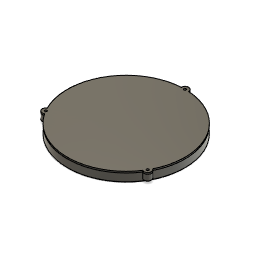
charging_base (Autodesk Fusion 360 design; units mm, degrees)
Autodesk Fusion 360 part; units mm, degrees
sketch "Sketch1" plane through (0, 0, 0) normal (0, 1, 0) x (1, 0, 0)
  circle A0 centre (0, 0) radius 65
  dimension "d1" = 130
  constraint coincident A0.centre origin
  measures "d1" diameter of A0
extrude "Extrude1" add sketch "Sketch1" along normal blind 1.6 makes body 1
sketch "Sketch2" plane through (0, 1.6, 0) normal (0, 1, 0) x (-1, 0, 0)
  circle A0 centre (0, 0) radius 65
  circle A1 centre (0, 0) radius 65
  circle A2 centre (0, 0) radius 62.5
  dimension "d4" = 130
  dimension "d5" = 125
  constraint coincident A0.centre A1.centre
  measures "d4" diameter of A1
  measures "d5" diameter of A2
extrude "Extrude2" add sketch "Sketch2" along normal blind 6.2 bodies 1
sketch "Sketch3" plane through (0, 1.6, 0) normal (0, 1, 0) x (-1, 0, 0)
  circle A0 centre (0, 0) radius 62.5
  circle A1 centre (0, 0) radius 20
  line L0 (0, 0) -> (0.5, 0)
  line L1 (0.5, 0) -> (-0.5, 0)
  circle A2 centre (0, 0) radius 62.5
  line L2 (-0.5, -47.9974) -> (-0.5, -62.498)
  line L3 (0.5, -62.498) -> (0.5, -47.9974)
  line L4 (0.5, -46.9973) -> (0.5, -33.9963)
  line L5 (0.5, -32.9962) -> (0.5, -20.994)
  line L6 (-0.5, -20.994) -> (-0.5, -32.9962)
  line L7 (-0.5, -33.9963) -> (-0.5, -46.9973)
  arc A3 (0.5, -47.9974) -> (23.5657, -41.817) centre (0, 0) ccw
  arc A4 (0.5, -46.9973) -> (23.0657, -40.9509) centre (0, 0) ccw
  line L8 (31.682, -53.8749) -> (24.4317, -41.317)
  line L9 (23.5657, -41.817) -> (30.816, -54.3749)
  arc A5 (0.5, -33.9963) -> (16.5651, -29.6917) centre (0, 0) ccw
  arc A6 (0.5, -32.9962) -> (16.0651, -28.8256) centre (0, 0) ccw
  line L10 (23.9317, -40.4509) -> (17.4312, -29.1917)
  line L11 (16.9311, -28.3256) -> (10.93, -17.9314)
  line L12 (10.064, -18.4314) -> (16.0651, -28.8256)
  line L13 (16.5651, -29.6917) -> (23.0657, -40.9509)
  arc A7 (0.5, -20.994) -> (10.064, -18.4314) centre (0, 0) ccw
  arc A8 (-10.064, -18.4314) -> (-0.5, -20.994) centre (0, 0) ccw
  arc A9 (-16.0651, -28.8256) -> (-0.5, -32.9962) centre (0, 0) ccw
  arc A10 (-16.5651, -29.6917) -> (-0.5, -33.9963) centre (0, 0) ccw
  line L14 (-16.0651, -28.8256) -> (-10.064, -18.4314)
  line L15 (-10.93, -17.9314) -> (-16.9311, -28.3256)
  arc A11 (-23.0657, -40.9509) -> (-0.5, -46.9973) centre (0, 0) ccw
  arc A12 (-23.5657, -41.817) -> (-0.5, -47.9974) centre (0, 0) ccw
  line L16 (-30.816, -54.3749) -> (-23.5657, -41.817)
  line L17 (-23.0657, -40.9509) -> (-16.5651, -29.6917)
  line L18 (-17.4312, -29.1917) -> (-23.9317, -40.4509)
  line L19 (-24.4317, -41.317) -> (-31.682, -53.8749)
  line L20 (41.317, -24.4317) -> (53.8749, -31.682)
  arc A13 (23.9317, -40.4509) -> (40.4509, -23.9317) centre (0, 0) ccw
  arc A14 (24.4317, -41.317) -> (41.317, -24.4317) centre (0, 0) ccw
  line L21 (54.3749, -30.816) -> (41.817, -23.5657)
  line L22 (17.9314, -10.93) -> (28.3256, -16.9311)
  line L23 (29.1917, -17.4312) -> (40.4509, -23.9317)
  line L24 (40.9509, -23.0657) -> (29.6917, -16.5651)
  line L25 (28.8256, -16.0651) -> (18.4314, -10.064)
  arc A15 (16.9311, -28.3256) -> (28.3256, -16.9311) centre (0, 0) ccw
  arc A16 (17.4312, -29.1917) -> (29.1917, -17.4312) centre (0, 0) ccw
  arc A17 (10.93, -17.9314) -> (17.9314, -10.93) centre (0, 0) ccw
  arc A18 (18.4314, -10.064) -> (20.994, -0.5) centre (0, 0) ccw
  arc A19 (28.8256, -16.0651) -> (32.9962, -0.5) centre (0, 0) ccw
  arc A20 (29.6917, -16.5651) -> (33.9963, -0.5) centre (0, 0) ccw
  arc A21 (40.9509, -23.0657) -> (46.9973, -0.5) centre (0, 0) ccw
  arc A22 (41.817, -23.5657) -> (47.9974, -0.5) centre (0, 0) ccw
  arc A23 (20.994, 0.5) -> (18.4314, 10.064) centre (0, 0) ccw
  arc A24 (32.9962, 0.5) -> (28.8256, 16.0651) centre (0, 0) ccw
  arc A25 (33.9963, 0.5) -> (29.6917, 16.5651) centre (0, 0) ccw
  arc A26 (46.9973, 0.5) -> (40.9509, 23.0657) centre (0, 0) ccw
  arc A27 (47.9974, 0.5) -> (41.817, 23.5657) centre (0, 0) ccw
  line L26 (20.994, -0.5) -> (32.9962, -0.5)
  line L27 (32.9962, 0.5) -> (20.994, 0.5)
  line L28 (33.9963, -0.5) -> (46.9973, -0.5)
  line L29 (47.9974, -0.5) -> (62.498, -0.5)
  line L30 (62.498, 0.5) -> (47.9974, 0.5)
  line L31 (46.9973, 0.5) -> (33.9963, 0.5)
  line L32 (18.4314, 10.064) -> (28.8256, 16.0651)
  line L33 (28.3256, 16.9311) -> (17.9314, 10.93)
  line L34 (29.6917, 16.5651) -> (40.9509, 23.0657)
  line L35 (41.817, 23.5657) -> (54.3749, 30.816)
  line L36 (53.8749, 31.682) -> (41.317, 24.4317)
  line L37 (40.4509, 23.9317) -> (29.1917, 17.4312)
  arc A28 (17.9314, 10.93) -> (10.93, 17.9314) centre (0, 0) ccw
  arc A29 (28.3256, 16.9311) -> (16.9311, 28.3256) centre (0, 0) ccw
  arc A30 (29.1917, 17.4312) -> (17.4312, 29.1917) centre (0, 0) ccw
  arc A31 (40.4509, 23.9317) -> (23.9317, 40.4509) centre (0, 0) ccw
  arc A32 (41.317, 24.4317) -> (24.4317, 41.317) centre (0, 0) ccw
  arc A33 (10.064, 18.4314) -> (0.5, 20.994) centre (0, 0) ccw
  arc A34 (16.0651, 28.8256) -> (0.5, 32.9962) centre (0, 0) ccw
  arc A35 (16.5651, 29.6917) -> (0.5, 33.9963) centre (0, 0) ccw
  arc A36 (23.0657, 40.9509) -> (0.5, 46.9973) centre (0, 0) ccw
  arc A37 (23.5657, 41.817) -> (0.5, 47.9974) centre (0, 0) ccw
  line L38 (10.93, 17.9314) -> (16.9311, 28.3256)
  line L39 (16.0651, 28.8256) -> (10.064, 18.4314)
  line L40 (17.4312, 29.1917) -> (23.9317, 40.4509)
  line L41 (24.4317, 41.317) -> (31.682, 53.8749)
  line L42 (30.816, 54.3749) -> (23.5657, 41.817)
  line L43 (23.0657, 40.9509) -> (16.5651, 29.6917)
  line L44 (0.5, 20.994) -> (0.5, 32.9962)
  line L45 (-0.5, 32.9962) -> (-0.5, 20.994)
  line L46 (0.5, 33.9963) -> (0.5, 46.9973)
  line L47 (0.5, 47.9974) -> (0.5, 62.498)
  line L48 (-0.5, 62.498) -> (-0.5, 47.9974)
  line L49 (-0.5, 46.9973) -> (-0.5, 33.9963)
  arc A38 (-0.5, 20.994) -> (-10.064, 18.4314) centre (0, 0) ccw
  arc A39 (-0.5, 32.9962) -> (-16.0651, 28.8256) centre (0, 0) ccw
  arc A40 (-0.5, 33.9963) -> (-16.5651, 29.6917) centre (0, 0) ccw
  arc A41 (-0.5, 46.9973) -> (-23.0657, 40.9509) centre (0, 0) ccw
  arc A42 (-0.5, 47.9974) -> (-23.5657, 41.817) centre (0, 0) ccw
  line L50 (-10.064, 18.4314) -> (-16.0651, 28.8256)
  line L51 (-16.9311, 28.3256) -> (-10.93, 17.9314)
  line L52 (-16.5651, 29.6917) -> (-23.0657, 40.9509)
  line L53 (-23.5657, 41.817) -> (-30.816, 54.3749)
  line L54 (-31.682, 53.8749) -> (-24.4317, 41.317)
  line L55 (-23.9317, 40.4509) -> (-17.4312, 29.1917)
  arc A43 (-10.93, 17.9314) -> (-17.9314, 10.93) centre (0, 0) ccw
  arc A44 (-16.9311, 28.3256) -> (-28.3256, 16.9311) centre (0, 0) ccw
  arc A45 (-17.4312, 29.1917) -> (-29.1917, 17.4312) centre (0, 0) ccw
  arc A46 (-23.9317, 40.4509) -> (-40.4509, 23.9317) centre (0, 0) ccw
  arc A47 (-24.4317, 41.317) -> (-41.317, 24.4317) centre (0, 0) ccw
  line L56 (-17.9314, 10.93) -> (-28.3256, 16.9311)
  line L57 (-28.8256, 16.0651) -> (-18.4314, 10.064)
  line L58 (-29.1917, 17.4312) -> (-40.4509, 23.9317)
  line L59 (-41.317, 24.4317) -> (-53.8749, 31.682)
  line L60 (-54.3749, 30.816) -> (-41.817, 23.5657)
  line L61 (-40.9509, 23.0657) -> (-29.6917, 16.5651)
  arc A48 (-18.4314, 10.064) -> (-20.994, 0.5) centre (0, 0) ccw
  arc A49 (-28.8256, 16.0651) -> (-32.9962, 0.5) centre (0, 0) ccw
  arc A50 (-29.6917, 16.5651) -> (-33.9963, 0.5) centre (0, 0) ccw
  arc A51 (-40.9509, 23.0657) -> (-46.9973, 0.5) centre (0, 0) ccw
  arc A52 (-41.817, 23.5657) -> (-47.9974, 0.5) centre (0, 0) ccw
  line L62 (-20.994, 0.5) -> (-32.9962, 0.5)
  line L63 (-32.9962, -0.5) -> (-20.994, -0.5)
  line L64 (-33.9963, 0.5) -> (-46.9973, 0.5)
  line L65 (-47.9974, 0.5) -> (-62.498, 0.5)
  line L66 (-62.498, -0.5) -> (-47.9974, -0.5)
  line L67 (-46.9973, -0.5) -> (-33.9963, -0.5)
  arc A53 (-20.994, -0.5) -> (-18.4314, -10.064) centre (0, 0) ccw
  arc A54 (-17.9314, -10.93) -> (-10.93, -17.9314) centre (0, 0) ccw
  arc A55 (-32.9962, -0.5) -> (-28.8256, -16.0651) centre (0, 0) ccw
  arc A56 (-28.3256, -16.9311) -> (-16.9311, -28.3256) centre (0, 0) ccw
  arc A57 (-33.9963, -0.5) -> (-29.6917, -16.5651) centre (0, 0) ccw
  arc A58 (-29.1917, -17.4312) -> (-17.4312, -29.1917) centre (0, 0) ccw
  arc A59 (-46.9973, -0.5) -> (-40.9509, -23.0657) centre (0, 0) ccw
  arc A60 (-40.4509, -23.9317) -> (-23.9317, -40.4509) centre (0, 0) ccw
  arc A61 (-47.9974, -0.5) -> (-41.817, -23.5657) centre (0, 0) ccw
  arc A62 (-41.317, -24.4317) -> (-24.4317, -41.317) centre (0, 0) ccw
  line L68 (-18.4314, -10.064) -> (-28.8256, -16.0651)
  line L69 (-28.3256, -16.9311) -> (-17.9314, -10.93)
  line L70 (-53.8749, -31.682) -> (-41.317, -24.4317)
  line L71 (-40.4509, -23.9317) -> (-29.1917, -17.4312)
  line L72 (-29.6917, -16.5651) -> (-40.9509, -23.0657)
  line L73 (-41.817, -23.5657) -> (-54.3749, -30.816)
  dimension "d8" = 40
  dimension "d9" = 42
  dimension "d10" = 0.5
  dimension "d11" = 1
  dimension "d15" = 125
  dimension "d16" = 66
  dimension "d17" = 68
  dimension "d18" = 94
  dimension "d19" = 96
  constraint coincident A0.centre A1.centre
  constraint horizontal L0
  constraint horizontal L1
  constraint vertical L6
  constraint vertical L3
  constraint coincident A0 L8.start
  constraint coincident A0 L9.end
  constraint coincident A0 L3.start
  constraint coincident A0 L2.end
  constraint coincident A0 L16.start
  constraint coincident A0 L19.end
  constraint coincident A0 L70.start
  constraint coincident A0 L73.end
  constraint coincident A0 L66.start
  constraint coincident A0 L65.end
  constraint coincident A0 L59.end
  constraint coincident A0 L60.start
  constraint coincident A0 L20.end
  constraint coincident A0 L21.start
  constraint coincident A0 L29.end
  constraint coincident A0 L30.start
  constraint coincident A0 L35.end
  constraint coincident A0 L36.start
  constraint coincident A0 L41.end
  constraint coincident A0 L42.start
  constraint coincident A0 L47.end
  constraint coincident A0 L48.start
  constraint coincident A0 L53.end
  constraint coincident A0 L54.start
  constraint coincident L2.start L6
  constraint coincident L4.start L3
  constraint collinear L2 L6
  constraint collinear L3 L4
  constraint coincident L7.start L6
  constraint collinear L4 L5
  constraint collinear L6 L7
  constraint coincident A3.end L12
  constraint concentric A3 A14
  constraint coincident L10.start L8
  constraint concentric A4 A13
  constraint collinear L8 L10
  constraint collinear L9 L12
  constraint coincident A5.end L12
  constraint concentric A5 A16
  constraint coincident L11.start L10
  constraint concentric A6 A15
  constraint collinear L10 L11
  constraint collinear L12 L13
  constraint concentric A7 A17
  constraint concentric A8 A17
  constraint coincident A9.start L16
  constraint concentric A9 A15
  constraint coincident L18.start L15
  constraint concentric A10 A16
  constraint collinear L14 L16
  constraint collinear L15 L18
  constraint coincident A11.start L16
  constraint concentric A11 A13
  constraint coincident L19.start L18
  constraint concentric A12 A14
  constraint collinear L16 L17
  constraint collinear L18 L19
  constraint collinear L20 L22
  constraint coincident L24.start L21
  constraint concentric A13 A21
  constraint concentric A14 A22
  constraint collinear L21 L24
  constraint collinear L22 L23
  constraint coincident L24.end A16
  constraint coincident L25.start A15
  constraint collinear L24 L25
  constraint concentric A15 A19
  constraint concentric A16 A20
  constraint concentric A17 A18
  constraint concentric A18 A23
  constraint coincident A24.start L30
  constraint concentric A19 A24
  constraint coincident A20.end L26
  constraint concentric A20 A25
  constraint coincident A21.end L26
  constraint coincident A26.start L30
  constraint concentric A21 A26
  constraint coincident A22.end L26
  constraint concentric A22 A27
  constraint concentric A23 A28
  constraint coincident L33.start L36
  constraint concentric A24 A29
  constraint coincident A25.end L32
  constraint concentric A25 A30
  constraint coincident A26.end L32
  constraint coincident L37.start L36
  constraint concentric A26 A31
  constraint coincident A27.end L32
  constraint concentric A27 A32
  constraint collinear L26 L28
  constraint collinear L27 L30
  constraint collinear L28 L29
  constraint collinear L30 L31
  constraint collinear L32 L34
  constraint collinear L33 L36
  constraint collinear L34 L35
  constraint collinear L36 L37
  constraint concentric A28 A33
  constraint coincident A34.start L42
  constraint concentric A29 A34
  constraint coincident A30.end L38
  constraint concentric A30 A35
  constraint coincident A31.end L38
  constraint coincident A36.start L42
  constraint concentric A31 A36
  constraint coincident A32.end L38
  constraint concentric A32 A37
  constraint concentric A33 A38
  constraint coincident L45.start L48
  constraint concentric A34 A39
  constraint coincident A35.end L44
  constraint concentric A35 A40
  constraint coincident A36.end L44
  constraint coincident L49.start L48
  constraint concentric A36 A41
  constraint coincident A37.end L44
  constraint concentric A37 A42
  constraint collinear L38 L40
  constraint collinear L39 L42
  constraint collinear L40 L41
  constraint collinear L42 L43
  constraint collinear L44 L46
  constraint collinear L45 L48
  constraint collinear L46 L47
  constraint collinear L48 L49
  constraint concentric A38 A43
  constraint coincident L51.start L54
  constraint concentric A39 A44
  constraint coincident A40.end L50
  constraint concentric A40 A45
  constraint coincident A41.end L50
  constraint coincident L55.start L54
  constraint concentric A41 A46
  constraint coincident A42.end L50
  constraint concentric A42 A47
  constraint collinear L50 L52
  constraint collinear L51 L54
  constraint collinear L52 L53
  constraint collinear L54 L55
  constraint concentric A43 A48
  constraint coincident L57.start L60
  constraint concentric A44 A49
  constraint coincident A45.end L56
  constraint concentric A45 A50
  constraint coincident A46.end L56
  constraint coincident L61.start L60
  constraint concentric A46 A51
  constraint coincident A47.end L56
  constraint concentric A47 A52
  constraint collinear L56 L58
  constraint collinear L57 L60
  constraint collinear L58 L59
  constraint collinear L60 L61
  constraint concentric A48 A53
  constraint coincident L63.start L66
  constraint concentric A49 A55
  constraint coincident A50.end L62
  constraint concentric A50 A57
  constraint coincident A51.end L62
  constraint coincident L67.start L66
  constraint concentric A51 A59
  constraint coincident A52.end L62
  constraint concentric A52 A61
  constraint collinear L62 L64
  constraint collinear L63 L66
  constraint collinear L64 L65
  constraint collinear L66 L67
  constraint concentric A53 A54
  constraint coincident A56.start L70
  constraint concentric A55 A56
  constraint coincident A57.end L68
  constraint concentric A57 A58
  constraint coincident A59.end L68
  constraint coincident A60.start L70
  constraint concentric A59 A60
  constraint coincident A61.end L68
  constraint concentric A61 A62
  constraint collinear L68 L72
  constraint collinear L69 L70
  constraint collinear L70 L71
  constraint collinear L72 L73
  measures "d8" diameter of A1
  measures "d9" diameter of A7
  measures "d10" distance of A0.centre L0.end
  measures "d11" distance of L0.end L1.end
  measures "d15" diameter of A2
  measures "d16" diameter of A6
  measures "d17" diameter of A5
  measures "d18" diameter of A4
  measures "d19" diameter of A3
extrude "Extrude3" add sketch "Sketch3" along normal blind 5.2 contours A0 A2 L2 L3 A3 L8 L9 A12 L16 L19 L20 A14 L21 A22 A27 L29 L30 L35 L36 A32 A37 L41 L42 L47 L48 A42 L53 L54 A47 L59 L60 A52 L65 L66 A61 A62 L70 L73 bodies 1
sketch "Sketch4" plane through (0, 6.8, 0) normal (0, 1, 0) x (-1, 0, 0)
  arc A0 (-40.9509, 23.0657) -> (-46.9973, 0.5) centre (0, 0) ccw
  line L0 (-40.9509, 23.0657) -> (-29.6917, 16.5651)
  arc A1 (-29.6917, 16.5651) -> (-33.9963, 0.5) centre (0, 0) ccw
  line L1 (-33.9963, 0.5) -> (-46.9973, 0.5)
  arc A2 (0.5, -46.9973) -> (23.0657, -40.9509) centre (0, 0) ccw
  line L2 (0.5, -46.9973) -> (0.5, -33.9963)
  arc A3 (0.5, -33.9963) -> (16.5651, -29.6917) centre (0, 0) ccw
  line L3 (16.5651, -29.6917) -> (23.0657, -40.9509)
  arc A4 (-16.0651, -28.8256) -> (-0.5, -32.9962) centre (0, 0) ccw
  line L4 (-16.0651, -28.8256) -> (-10.064, -18.4314)
  arc A5 (-10.064, -18.4314) -> (-0.5, -20.994) centre (0, 0) ccw
  line L5 (-0.5, -20.994) -> (-0.5, -32.9962)
  arc A6 (28.3256, 16.9311) -> (16.9311, 28.3256) centre (0, 0) ccw
  line L6 (28.3256, 16.9311) -> (17.9314, 10.93)
  arc A7 (17.9314, 10.93) -> (10.93, 17.9314) centre (0, 0) ccw
  line L7 (10.93, 17.9314) -> (16.9311, 28.3256)
  arc A8 (23.0657, 40.9509) -> (0.5, 46.9973) centre (0, 0) ccw
  line L8 (23.0657, 40.9509) -> (16.5651, 29.6917)
  arc A9 (16.5651, 29.6917) -> (0.5, 33.9963) centre (0, 0) ccw
  line L9 (0.5, 33.9963) -> (0.5, 46.9973)
  circle A10 centre (0, 0) radius 20
  arc A11 (-0.5, 32.9962) -> (-16.0651, 28.8256) centre (0, 0) ccw
  line L10 (-0.5, 32.9962) -> (-0.5, 20.994)
  arc A12 (-0.5, 20.994) -> (-10.064, 18.4314) centre (0, 0) ccw
  line L11 (-10.064, 18.4314) -> (-16.0651, 28.8256)
  arc A13 (-46.9973, -0.5) -> (-40.9509, -23.0657) centre (0, 0) ccw
  line L12 (-46.9973, -0.5) -> (-33.9963, -0.5)
  arc A14 (-33.9963, -0.5) -> (-29.6917, -16.5651) centre (0, 0) ccw
  line L13 (-29.6917, -16.5651) -> (-40.9509, -23.0657)
  arc A15 (-23.9317, 40.4509) -> (-40.4509, 23.9317) centre (0, 0) ccw
  line L14 (-23.9317, 40.4509) -> (-17.4312, 29.1917)
  arc A16 (-17.4312, 29.1917) -> (-29.1917, 17.4312) centre (0, 0) ccw
  line L15 (-29.1917, 17.4312) -> (-40.4509, 23.9317)
  arc A17 (-40.4509, -23.9317) -> (-23.9317, -40.4509) centre (0, 0) ccw
  line L16 (-40.4509, -23.9317) -> (-29.1917, -17.4312)
  arc A18 (-29.1917, -17.4312) -> (-17.4312, -29.1917) centre (0, 0) ccw
  line L17 (-17.4312, -29.1917) -> (-23.9317, -40.4509)
  arc A19 (-23.0657, -40.9509) -> (-0.5, -46.9973) centre (0, 0) ccw
  line L18 (-23.0657, -40.9509) -> (-16.5651, -29.6917)
  arc A20 (-16.5651, -29.6917) -> (-0.5, -33.9963) centre (0, 0) ccw
  line L19 (-0.5, -33.9963) -> (-0.5, -46.9973)
  arc A21 (0.5, -32.9962) -> (16.0651, -28.8256) centre (0, 0) ccw
  line L20 (0.5, -32.9962) -> (0.5, -20.994)
  arc A22 (0.5, -20.994) -> (10.064, -18.4314) centre (0, 0) ccw
  line L21 (10.064, -18.4314) -> (16.0651, -28.8256)
  arc A23 (-0.5, 46.9973) -> (-23.0657, 40.9509) centre (0, 0) ccw
  line L22 (-0.5, 46.9973) -> (-0.5, 33.9963)
  arc A24 (-0.5, 33.9963) -> (-16.5651, 29.6917) centre (0, 0) ccw
  line L23 (-16.5651, 29.6917) -> (-23.0657, 40.9509)
  arc A25 (40.4509, 23.9317) -> (23.9317, 40.4509) centre (0, 0) ccw
  line L24 (40.4509, 23.9317) -> (29.1917, 17.4312)
  arc A26 (29.1917, 17.4312) -> (17.4312, 29.1917) centre (0, 0) ccw
  line L25 (17.4312, 29.1917) -> (23.9317, 40.4509)
  arc A27 (16.0651, 28.8256) -> (0.5, 32.9962) centre (0, 0) ccw
  line L26 (16.0651, 28.8256) -> (10.064, 18.4314)
  arc A28 (10.064, 18.4314) -> (0.5, 20.994) centre (0, 0) ccw
  line L27 (0.5, 20.994) -> (0.5, 32.9962)
  arc A29 (-32.9962, -0.5) -> (-28.8256, -16.0651) centre (0, 0) ccw
  line L28 (-32.9962, -0.5) -> (-20.994, -0.5)
  arc A30 (-20.994, -0.5) -> (-18.4314, -10.064) centre (0, 0) ccw
  line L29 (-18.4314, -10.064) -> (-28.8256, -16.0651)
  arc A31 (-28.8256, 16.0651) -> (-32.9962, 0.5) centre (0, 0) ccw
  line L30 (-28.8256, 16.0651) -> (-18.4314, 10.064)
  arc A32 (-18.4314, 10.064) -> (-20.994, 0.5) centre (0, 0) ccw
  line L31 (-20.994, 0.5) -> (-32.9962, 0.5)
  arc A33 (-16.9311, 28.3256) -> (-28.3256, 16.9311) centre (0, 0) ccw
  line L32 (-16.9311, 28.3256) -> (-10.93, 17.9314)
  arc A34 (-10.93, 17.9314) -> (-17.9314, 10.93) centre (0, 0) ccw
  line L33 (-17.9314, 10.93) -> (-28.3256, 16.9311)
  arc A35 (23.9317, -40.4509) -> (40.4509, -23.9317) centre (0, 0) ccw
  line L34 (23.9317, -40.4509) -> (17.4312, -29.1917)
  arc A36 (17.4312, -29.1917) -> (29.1917, -17.4312) centre (0, 0) ccw
  line L35 (29.1917, -17.4312) -> (40.4509, -23.9317)
  arc A37 (16.9311, -28.3256) -> (28.3256, -16.9311) centre (0, 0) ccw
  line L36 (16.9311, -28.3256) -> (10.93, -17.9314)
  arc A38 (10.93, -17.9314) -> (17.9314, -10.93) centre (0, 0) ccw
  line L37 (17.9314, -10.93) -> (28.3256, -16.9311)
  arc A39 (-28.3256, -16.9311) -> (-16.9311, -28.3256) centre (0, 0) ccw
  line L38 (-28.3256, -16.9311) -> (-17.9314, -10.93)
  arc A40 (-17.9314, -10.93) -> (-10.93, -17.9314) centre (0, 0) ccw
  line L39 (-10.93, -17.9314) -> (-16.9311, -28.3256)
  arc A41 (46.9973, 0.5) -> (40.9509, 23.0657) centre (0, 0) ccw
  line L40 (46.9973, 0.5) -> (33.9963, 0.5)
  arc A42 (33.9963, 0.5) -> (29.6917, 16.5651) centre (0, 0) ccw
  line L41 (29.6917, 16.5651) -> (40.9509, 23.0657)
  arc A43 (32.9962, 0.5) -> (28.8256, 16.0651) centre (0, 0) ccw
  line L42 (32.9962, 0.5) -> (20.994, 0.5)
  arc A44 (20.994, 0.5) -> (18.4314, 10.064) centre (0, 0) ccw
  line L43 (18.4314, 10.064) -> (28.8256, 16.0651)
  arc A45 (28.8256, -16.0651) -> (32.9962, -0.5) centre (0, 0) ccw
  line L44 (28.8256, -16.0651) -> (18.4314, -10.064)
  arc A46 (18.4314, -10.064) -> (20.994, -0.5) centre (0, 0) ccw
  line L45 (20.994, -0.5) -> (32.9962, -0.5)
  arc A47 (40.9509, -23.0657) -> (46.9973, -0.5) centre (0, 0) ccw
  line L46 (40.9509, -23.0657) -> (29.6917, -16.5651)
  arc A48 (29.6917, -16.5651) -> (33.9963, -0.5) centre (0, 0) ccw
  line L47 (33.9963, -0.5) -> (46.9973, -0.5)
  line L48 (-41.817, -23.5657) -> (-54.3749, -30.816)
  arc A49 (-54.3749, -30.816) -> (-53.8749, -31.682) centre (0, 0) ccw
  line L49 (-53.8749, -31.682) -> (-41.317, -24.4317)
  arc A50 (-41.317, -24.4317) -> (-24.4317, -41.317) centre (0, 0) ccw
  line L50 (-24.4317, -41.317) -> (-31.682, -53.8749)
  arc A51 (-31.682, -53.8749) -> (-30.816, -54.3749) centre (0, 0) ccw
  line L51 (-30.816, -54.3749) -> (-23.5657, -41.817)
  arc A52 (-23.5657, -41.817) -> (-0.5, -47.9974) centre (0, 0) ccw
  line L52 (-0.5, -47.9974) -> (-0.5, -62.498)
  arc A53 (-0.5, -62.498) -> (0.5, -62.498) centre (0, 0) ccw
  line L53 (0.5, -62.498) -> (0.5, -47.9974)
  arc A54 (0.5, -47.9974) -> (23.5657, -41.817) centre (0, 0) ccw
  line L54 (23.5657, -41.817) -> (30.816, -54.3749)
  arc A55 (30.816, -54.3749) -> (31.682, -53.8749) centre (0, 0) ccw
  line L55 (31.682, -53.8749) -> (24.4317, -41.317)
  arc A56 (24.4317, -41.317) -> (41.317, -24.4317) centre (0, 0) ccw
  line L56 (41.317, -24.4317) -> (53.8749, -31.682)
  arc A57 (53.8749, -31.682) -> (54.3749, -30.816) centre (0, 0) ccw
  line L57 (54.3749, -30.816) -> (41.817, -23.5657)
  arc A58 (41.817, -23.5657) -> (47.9974, -0.5) centre (0, 0) ccw
  line L58 (47.9974, -0.5) -> (62.498, -0.5)
  arc A59 (62.498, -0.5) -> (62.498, 0.5) centre (0, 0) ccw
  line L59 (62.498, 0.5) -> (47.9974, 0.5)
  arc A60 (47.9974, 0.5) -> (41.817, 23.5657) centre (0, 0) ccw
  line L60 (41.817, 23.5657) -> (54.3749, 30.816)
  arc A61 (54.3749, 30.816) -> (53.8749, 31.682) centre (0, 0) ccw
  line L61 (53.8749, 31.682) -> (41.317, 24.4317)
  arc A62 (41.317, 24.4317) -> (24.4317, 41.317) centre (0, 0) ccw
  line L62 (24.4317, 41.317) -> (31.682, 53.8749)
  arc A63 (31.682, 53.8749) -> (30.816, 54.3749) centre (0, 0) ccw
  line L63 (30.816, 54.3749) -> (23.5657, 41.817)
  arc A64 (23.5657, 41.817) -> (0.5, 47.9974) centre (0, 0) ccw
  line L64 (0.5, 47.9974) -> (0.5, 62.498)
  arc A65 (0.5, 62.498) -> (-0.5, 62.498) centre (0, 0) ccw
  line L65 (-0.5, 62.498) -> (-0.5, 47.9974)
  arc A66 (-0.5, 47.9974) -> (-23.5657, 41.817) centre (0, 0) ccw
  line L66 (-23.5657, 41.817) -> (-30.816, 54.3749)
  arc A67 (-30.816, 54.3749) -> (-31.682, 53.8749) centre (0, 0) ccw
  line L67 (-31.682, 53.8749) -> (-24.4317, 41.317)
  arc A68 (-24.4317, 41.317) -> (-41.317, 24.4317) centre (0, 0) ccw
  line L68 (-41.317, 24.4317) -> (-53.8749, 31.682)
  arc A69 (-53.8749, 31.682) -> (-54.3749, 30.816) centre (0, 0) ccw
  line L69 (-54.3749, 30.816) -> (-41.817, 23.5657)
  arc A70 (-41.817, 23.5657) -> (-47.9974, 0.5) centre (0, 0) ccw
  line L70 (-47.9974, 0.5) -> (-62.498, 0.5)
  arc A71 (-62.498, 0.5) -> (-62.498, -0.5) centre (0, 0) ccw
  line L71 (-62.498, -0.5) -> (-47.9974, -0.5)
  arc A72 (-47.9974, -0.5) -> (-41.817, -23.5657) centre (0, 0) ccw
  circle A73 centre (0, 0) radius 47.5
  line L72 (0, 0) -> (75, 0)
  circle A74 centre (47.5, 0) radius 1
  circle A75 centre (0, 47.5) radius 1
  circle A76 centre (-47.5, 0) radius 1
  circle A77 centre (0, -47.5) radius 1
  point P0 (0.5, 47.9974)
  point P1 (-47.9974, 0.5)
  point P2 (-0.5, -47.9974)
  dimension "d22" = 95
  dimension "d23" = 75
  dimension "d24" = 2
  dimension "d26" = 360
  constraint coincident A0.centre A1.centre
  constraint horizontal L72
  constraint coincident L72 A74.centre
  constraint coincident A73 A74.centre
  measures "d22" diameter of A73
  measures "d23" distance of A0.centre L72.end
  measures "d24" diameter of A74
extrude "Extrude4" add sketch "Sketch4" along normal blind 1 contours A0 L1 A13 L12 A73 A76 | A70 L70 L71 A72 A73 A76 | A64 L64 L65 A66 A73 A75 | A8 L9 A23 L22 A73 A75 | A2 L2 A19 L19 A73 A77 | A52 L52 L53 A54 A73 A77 | L59 A60 A73 L72 A74 | A41 L40 A73 L72 A74 | A58 L58 A73 L72 A74 | A47 L47 A73 L72 A74 bodies 1
sketch "Sketch5" plane through (0, 7.8, 0) normal (0, 1, 0) x (-1, 0, 0)
  arc A0 (46.9921, -0.8614) -> (47.9921, -0.8705) centre (47.5, 0) ccw
  arc A1 (47.9921, -0.8705) -> (47.9974, -0.5) centre (0, 0) ccw
  line L0 (47.9974, -0.5) -> (48.366, -0.5)
  arc A2 (48.366, -0.5) -> (48.366, 0.5) centre (47.5, 0) ccw
  line L1 (48.366, 0.5) -> (47.9974, 0.5)
  arc A3 (47.9974, 0.5) -> (47.9921, 0.8705) centre (0, 0) ccw
  arc A4 (47.9921, 0.8705) -> (46.9921, 0.8614) centre (47.5, 0) ccw
  arc A5 (46.9973, 0.5) -> (46.9921, 0.8614) centre (0, 0) ccw
  line L2 (46.9973, 0.5) -> (46.634, 0.5)
  arc A6 (46.634, 0.5) -> (46.634, -0.5) centre (47.5, 0) ccw
  line L3 (46.634, -0.5) -> (46.9973, -0.5)
  arc A7 (46.9921, -0.8614) -> (46.9973, -0.5) centre (0, 0) ccw
  line L4 (0, 0) -> (70, 0)
  circle A8 centre (0, 0) radius 47.5
  circle A9 centre (47.5, 0) radius 0.675
  circle A10 centre (0, 47.5) radius 0.675
  circle A11 centre (-47.5, 0) radius 0.675
  circle A12 centre (0, -47.5) radius 0.675
  dimension "d29" = 70
  dimension "d30" = 95
  dimension "d31" = 1.35
  dimension "d33" = 360
  constraint coincident A1.centre A3.centre
  constraint horizontal L4
  constraint concentric A0 A9
  measures "d29" distance of A1.centre L4.end
  measures "d30" diameter of A8
  measures "d31" diameter of A9
extrude "Extrude5" add sketch "Sketch5" along normal blind 1 contours A8 A12 | A8 A12 | L4 A8 A9 | L4 A8 A9 | L4 A8 A9 | L4 A8 A9 | A8 A11 | A8 A11 | A8 A10 | A8 A10 bodies 1
sketch "Sketch6" plane through (0, 1.6, 0) normal (0, 1, 0) x (-1, 0, 0)
  circle A0 centre (0, 0) radius 20
  line L0 (-7, 3) -> (7, 3)
  line L1 (7, 3) -> (7, -3)
  line L2 (7, -3) -> (-7, -3)
  line L3 (-7, -3) -> (-7, 3)
  line L4 (-7, 3) -> (7, -3) construction
  line L5 (7, 3) -> (-7, -3) construction
  dimension "d36" = 14
  dimension "d37" = 6
  constraint perpendicular L0 L1
  constraint parallel L0 L2
  constraint parallel L1 L3
  constraint horizontal L0
  constraint coincident L4 A0.centre
  constraint coincident L5 A0.centre
  constraint coincident A0.centre origin
  measures "d36" distance of L1.end L2.end
  measures "d37" distance of L0.end L1.end
extrude "Extrude6" cut sketch "Sketch6" against normal blind 5 contours L0 L1 L2 L3 bodies 1
sketch "Sketch7" plane through (0, 1.6, 0) normal (0, 1, 0) x (-1, 0, 0)
  line L0 (7, 3) -> (7, -3)
  line L1 (7, -3) -> (-7, -3)
  line L2 (-7, -3) -> (-7, 3)
  line L3 (-7, 3) -> (7, 3)
  circle A0 centre (0, 0) radius 20
  line L4 (-8, -4) -> (8, -4)
  line L5 (8, -4) -> (8, 4)
  line L6 (8, 4) -> (-8, 4)
  line L7 (-8, 4) -> (-8, -4)
  line L8 (-8, -4) -> (8, 4) construction
  line L9 (8, -4) -> (-8, 4) construction
  dimension "d40" = 16
  dimension "d41" = 8
  constraint perpendicular L4 L5
  constraint parallel L4 L6
  constraint parallel L5 L7
  constraint horizontal L4
  constraint coincident L8 A0.centre
  constraint coincident L9 A0.centre
  constraint coincident A0.centre origin
  measures "d40" distance of L5.end L6.end
  measures "d41" distance of L4.end L5.end
extrude "Extrude7" add sketch "Sketch7" along normal blind 4.2 contours L4 L5 L6 L7 bodies 1
sketch "Sketch8" plane through (0, 5.8, 0) normal (0, 1, 0) x (-1, 0, 0)
  line L0 (-7, -3) -> (-7, 3)
  line L1 (-7, 3) -> (7, 3)
  line L2 (7, 3) -> (7, -3)
  line L3 (7, -3) -> (-7, -3)
  line L4 (-8, 4) -> (-8, -4)
  line L5 (-8, -4) -> (8, -4)
  line L6 (8, -4) -> (8, 4)
  line L7 (8, 4) -> (-8, 4)
  line L8 (-0.5, 3) -> (0.5, 3)
  line L9 (0.5, 3) -> (0.5, -3)
  line L10 (0.5, -3) -> (-0.5, -3)
  line L11 (-0.5, -3) -> (-0.5, 3)
  line L12 (-0.5, 3) -> (0.5, -3) construction
  line L13 (0.5, 3) -> (-0.5, -3) construction
  dimension "d44" = 1
  dimension "d45" = 6
  constraint perpendicular L8 L9
  constraint parallel L8 L10
  constraint parallel L9 L11
  constraint horizontal L8
  constraint coincident L12 origin
  constraint coincident L13 origin
  measures "d44" distance of L9.end L10.end
  measures "d45" distance of L8.end L9.end
extrude "Extrude8" add sketch "Sketch8" against normal blind 3.6 contours L1 L3 L8 L9 L10 L11 bodies 1
extrude "Extrude9" add 1 faces at (-63.692, 7.8, -6.3343) along direction (0, 1, 0) blind 1.6 on bodies 1 bodies 1
sketch "Sketch11" plane through (0, 9.4, 0) normal (0, 1, 0) x (-1, 0, 0)
  circle A0 centre (0, 0) radius 62.5
  circle A1 centre (0, 0) radius 65
  line L0 (56.5, -8) -> (73.5, -8)
  line L1 (73.5, -8) -> (73.5, 8)
  line L2 (73.5, 8) -> (56.5, 8)
  line L3 (56.5, 8) -> (56.5, -8)
  line L4 (56.5, -8) -> (73.5, 8) construction
  line L5 (73.5, -8) -> (56.5, 8) construction
  point P0 (65, 0)
  point P1 (65, 0)
  dimension "d57" = 17
  dimension "d58" = 16
  constraint perpendicular L0 L1
  constraint parallel L0 L2
  constraint parallel L1 L3
  constraint horizontal L0
  constraint coincident L4 P1
  constraint coincident L5 P1
  constraint coincident P1 P0
  measures "d57" distance of L1.end L2.end
  measures "d58" distance of L0.end L1.end
extrude "Extrude10" cut sketch "Sketch11" against normal blind 5.5 contours A0 L0 L2 L3 | A0 A1 L0 L2 | A1 L0 L1 L2 picked at (58.5, 0) picked at (62.921, -7.1138) bodies 1
fillet "Fillet1" radius 2.5 1 edges at (-56.5, 3.9, 0) on bodies 1
fillet "Fillet2" radius 2 2 edges at (-63.2458, 3.9, -8) (-63.2458, 3.9, 8) on bodies 1
sketch "Sketch12" plane through (0, 9.4, 0) normal (0, 1, 0) x (-1, 0, 0)
  line L0 (61.9859, 8) -> (64.5058, 8)
  arc A0 (64.5058, 8) -> (64.5058, -8) centre (0, 0) ccw
  line L1 (64.5058, -8) -> (61.9859, -8)
  arc A1 (61.9859, 8) -> (61.9859, -8) centre (0, 0) ccw
  circle A2 centre (0, -65) radius 4
  circle A3 centre (56.2917, 32.5) radius 4
  circle A4 centre (-56.2917, 32.5) radius 4
  dimension "d66" = 360
  dimension "d79" = 8
  constraint coincident A0 A2.centre
  measures "d79" diameter of A2
extrude "Extrude11" add sketch "Sketch12" against normal blind 7.4 contours A0 A3 | A0 A4 | A0 A2 bodies 1
sketch "Sketch13" plane through (0, 9.4, 0) normal (0, 1, 0) x (-1, 0, 0)
  line L0 (61.9859, 8) -> (64.5058, 8)
  arc A0 (64.5058, 8) -> (58.1841, 28.976) centre (0, 0) ccw
  arc A1 (58.1841, 28.976) -> (54.186, 35.9009) centre (56.2917, 32.5) ccw
  arc A2 (54.186, 35.9009) -> (-54.186, 35.9009) centre (0, 0) ccw
  arc A3 (-54.186, 35.9009) -> (-58.1841, 28.976) centre (-56.2917, 32.5) ccw
  arc A4 (-58.1841, 28.976) -> (-3.9981, -64.8769) centre (0, 0) ccw
  arc A5 (-3.9981, -64.8769) -> (3.9981, -64.8769) centre (0, -65) ccw
  arc A6 (3.9981, -64.8769) -> (64.5058, -8) centre (0, 0) ccw
  line L1 (64.5058, -8) -> (61.9859, -8)
  arc A7 (61.9859, 8) -> (61.9859, -8) centre (0, 0) ccw
  point P0 (0, -65)
  point P1 (56.2917, 32.5)
  point P2 (-56.2917, 32.5)
  constraint coincident P0 A5.centre
  constraint coincident P1 A1.centre
  constraint coincident P2 A3.centre
hole "Hole1" at (-56.2917, 9.4, 32.5) at (0, 9.4, -65) at (56.2917, 9.4, 32.5) direction (0, -1, 0) diameter 2.2 depth 6.4 tip angle 180 bodies 1
chamfer "Chamfer1" distance 1 angle 45 1 edges at (-60.6013, 0, 23.505) on bodies 1
chamfer "Chamfer2" distance 1 angle 45 3 edges at (0, 2, -69) (59.7558, 2, 34.5) (-59.7558, 2, 34.5) on bodies 1
sketch "Sketch15" plane through (0, 9.4, 0) normal (0, 1, 0) x (-1, 0, 0)
  circle A0 centre (0, -65) radius 1.1
  circle A1 centre (56.2917, 32.5) radius 1.1
  circle A2 centre (-56.2917, 32.5) radius 1.1
  line L0 (61.9859, 8) -> (64.5058, 8)
  arc A3 (64.5058, 8) -> (58.1841, 28.976) centre (0, 0) ccw
  arc A4 (58.1841, 28.976) -> (54.186, 35.9009) centre (56.2917, 32.5) ccw
  arc A5 (54.186, 35.9009) -> (-54.186, 35.9009) centre (0, 0) ccw
  arc A6 (-54.186, 35.9009) -> (-58.1841, 28.976) centre (-56.2917, 32.5) ccw
  arc A7 (-58.1841, 28.976) -> (-3.9981, -64.8769) centre (0, 0) ccw
  arc A8 (-3.9981, -64.8769) -> (3.9981, -64.8769) centre (0, -65) ccw
  arc A9 (3.9981, -64.8769) -> (64.5058, -8) centre (0, 0) ccw
  line L1 (64.5058, -8) -> (61.9859, -8)
  arc A10 (61.9859, 8) -> (61.9859, -8) centre (0, 0) ccw
  circle A11 centre (0, 0) radius 65
  constraint concentric A3 A11
extrude "Extrude12" add sketch "Sketch15" along normal blind 1.6 separate body makes body 2
sketch "Sketch16" plane through (0, 11, 0) normal (0, 1, 0) x (-1, 0, 0)
  arc A0 (-54.186, 35.9009) -> (-58.1841, 28.976) centre (-56.2917, 32.5) ccw
  arc A1 (-58.1841, 28.976) -> (-3.9981, -64.8769) centre (0, 0) ccw
  arc A2 (-3.9981, -64.8769) -> (3.9981, -64.8769) centre (0, -65) ccw
  arc A3 (3.9981, -64.8769) -> (58.1841, 28.976) centre (0, 0) ccw
  arc A4 (58.1841, 28.976) -> (54.186, 35.9009) centre (56.2917, 32.5) ccw
  arc A5 (54.186, 35.9009) -> (-54.186, 35.9009) centre (0, 0) ccw
  point P0 (0, -65)
  point P1 (56.2917, 32.5)
  point P2 (-56.2917, 32.5)
  constraint coincident P0 A2.centre
  constraint coincident P1 A4.centre
  constraint coincident P2 A0.centre
hole "Hole2" at (0, 11, -65) at (-56.2917, 11, 32.5) at (56.2917, 11, 32.5) direction (0, -1, 0) diameter 2.5 depth 1.6 tip angle 180 bodies 2
equation "d1 = 65 mm * 2"
